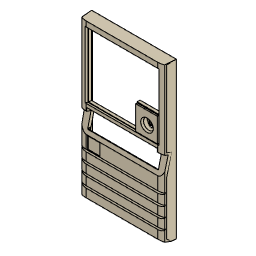
ks-330-front-1.0-dev (Autodesk Fusion 360 design; units mm, degrees)
Autodesk Fusion 360 part; units mm, degrees
sketch "Base-Front" plane through (0, 0, 0) normal (0, 1, 0) x (1, 0, 0)
  line L0 (-90, 0) -> (90, 0)
  line L1 (90, 0) -> (90, -330)
  line L2 (90, -330) -> (-90, -330)
  line L3 (-90, -330) -> (-90, 0)
  dimension "d1" = 180
  dimension "d2" = 330
  constraint horizontal L0
  constraint vertical L1
  constraint horizontal L2
  constraint vertical L3
  measures "d1" distance of L0.start L0.end
  measures "d2" distance of L0.start L2.end
extrude "Extrude1" add sketch "Base-Front" along normal blind 3.25 makes body 1
sketch "Back-OuterFrame" plane through (0, 3.25, 0) normal (0, 1, 0) x (-1, 0, 0)
  line L0 (90, 330) -> (-90, 330)
  line L1 (-90, 330) -> (-90, 0)
  line L2 (-90, 0) -> (90, 0)
  line L3 (90, 0) -> (90, 330)
  line L4 (-88, 328) -> (88, 328)
  line L5 (88, 328) -> (88, 2)
  line L6 (88, 2) -> (-88, 2)
  line L7 (-88, 2) -> (-88, 328)
  dimension "d5" = 2
  dimension "d6" = 2
  dimension "d7" = 2
  dimension "d8" = 2
  constraint horizontal L4
  constraint vertical L5
  constraint horizontal L6
  constraint vertical L7
  measures "d5" distance of L3 L5
  measures "d6" distance of L1 L7
  measures "d7" distance of L0 L4.end
  measures "d8" distance of L2 L6
sketch "Back-DriveBay" plane through (0, 3.25, 165) normal (0, 1, 0) x (-1, 0, 0)
  line L0 (-75, 153) -> (75, 153)
  line L1 (75, 153) -> (75, 14.5)
  line L2 (75, 14.5) -> (-75, 14.5)
  line L3 (-75, 14.5) -> (-75, 153)
  line L4 (-90, 165) -> (-90, -165)
  line L5 (90, -165) -> (90, 165)
  line L6 (-75, 153) -> (74.5, 153)
  line L7 (74.5, 153) -> (74.5, 109.75)
  line L8 (74.5, 109.75) -> (-75, 109.75)
  line L9 (-75, 109.75) -> (-75, 153)
  line L10 (-75, 109.75) -> (74.5, 109.75)
  line L11 (74.5, 109.75) -> (74.5, 66.5)
  line L12 (74.5, 66.5) -> (-75, 66.5)
  line L13 (-75, 66.5) -> (-75, 109.75)
  line L14 (-75, 66.5) -> (-28, 66.5)
  line L15 (-28, 66.5) -> (-28, 14.5)
  line L16 (-28, 14.5) -> (-75, 14.5)
  line L17 (-75, 14.5) -> (-75, 66.5)
  line L18 (74.5, 66.9726) -> (74.5, 40.5)
  line L19 (74.5, 40.5) -> (-28, 40.5)
  line L20 (-28, 40.5) -> (-28, 66.5)
  line L21 (-90, 165) -> (90, 165)
  dimension "d9" = 150
  dimension "d10" = 15
  dimension "d11" = 16
  dimension "d12" = 43.25
  dimension "d13" = 43.25
  dimension "d14" = 138.5
  dimension "d15" = 51.75
  dimension "d16" = 47
  dimension "d17" = 102.5
  dimension "d20" = 26
  dimension "d22" = 26
  dimension "d27" = 12
  constraint horizontal L0
  constraint vertical L1
  constraint horizontal L2
  constraint vertical L3
  constraint horizontal L6
  constraint vertical L7
  constraint horizontal L8
  constraint vertical L9
  constraint horizontal L10
  constraint vertical L11
  constraint horizontal L12
  constraint vertical L13
  constraint horizontal L14
  constraint vertical L15
  constraint horizontal L16
  constraint vertical L17
  constraint coincident L2 L15.end
  constraint vertical L18
  constraint horizontal L19
  constraint vertical L20
  measures "d9" distance of L1 L3
  measures "d10" distance of L3 L4
  measures "d12" distance of L0.start L8.end
  measures "d13" distance of L8.end L12.end
  measures "d14" distance of L2 L6
  measures "d16" distance of L15 L17
  measures "d20" distance of L14.end L19.end
  measures "d22" distance of L2 L19
  measures "d27" distance of L0 L21
sketch "Back-DriveBayFrame" plane through (0, 3.25, 165) normal (0, 1, 0) x (-1, 0, 0)
  line L0 (-79, 156) -> (79, 156)
  line L1 (79, 156) -> (79, 11.5)
  line L2 (79, 11.5) -> (-79, 11.5)
  line L3 (-79, 11.5) -> (-79, 156)
  line L4 (-75, 153) -> (74.5, 153)
  line L5 (75, 14.5) -> (-75, 14.5)
  line L6 (75, 153) -> (75, 14.5)
  line L7 (-75, 14.5) -> (-75, 153)
  line L8 (-75, 153) -> (75, 153)
  line L9 (75, 153) -> (75, 14.5)
  line L10 (75, 14.5) -> (-75, 14.5)
  line L11 (-75, 14.5) -> (-75, 153)
  line L12 (-79, 156) -> (79, 156)
  line L13 (-77, 155) -> (77, 155)
  line L14 (77, 155) -> (77, 12.5)
  line L15 (77, 12.5) -> (-30, 12.5)
  line L16 (-30, 12.5) -> (-30, 14.5)
  line L17 (-77, 155) -> (-77, 64.5)
  line L18 (-77, 64.5) -> (-75, 64.5)
  line L19 (-75, 64.5) -> (-30, 64.5)
  line L20 (-30, 64.5) -> (-30, 14.5)
  line L21 (74.5, 66.5) -> (-75, 66.5)
  line L22 (-28, 66.5) -> (-28, 14.5)
  line L23 (-75, 66.5) -> (-28, 66.5)
  line L24 (-28, 14.5) -> (75, 14.5)
  line L25 (-75, 66.5) -> (-75, 153)
  line L26 (75, 153) -> (75, 14.5)
  line L27 (-28, 66.5) -> (-28, 14.5)
  dimension "d23" = 3
  dimension "d24" = 3
  dimension "d25" = 4
  dimension "d26" = 4
  dimension "d29" = 2
  dimension "d30" = 2
  dimension "d32" = 2
  dimension "d33" = 107
  dimension "d34" = 2
  dimension "d35" = 2
  dimension "d36" = 90.5
  dimension "d39" = 2
  constraint horizontal L0
  constraint vertical L1
  constraint horizontal L2
  constraint vertical L3
  constraint horizontal L8
  constraint vertical L9
  constraint horizontal L10
  constraint vertical L11
  constraint coincident L5.start L6.end
  constraint coincident L4.start L7.end
  constraint perpendicular L3 L13
  constraint perpendicular L8 L14
  constraint perpendicular L14 L15
  constraint coincident L5 L16.end
  constraint perpendicular L5 L16
  constraint perpendicular L13 L17
  constraint coincident L7 L18.end
  constraint perpendicular L7 L18
  constraint perpendicular L11 L19
  constraint vertical L20
  constraint coincident L21.end L23.start
  constraint coincident L22.start L23.end
  constraint coincident L22.end L24.start
  constraint coincident L6.start L8.end
  measures "d23" distance of L0 L4
  measures "d24" distance of L2 L5
  measures "d25" distance of L1 L6
  measures "d26" distance of L3 L7
  measures "d29" distance of L11 L17
  measures "d30" distance of L8 L13
  measures "d32" distance of L10 L15
  measures "d33" distance of L14.end L15.end
  measures "d34" distance of L15.end L16.end
  measures "d35" distance of L6 L14
  measures "d36" distance of L13.start L17.end
  measures "d39" distance of L20 L22
sketch "Back-FrontPanel" plane through (0, 3.25, 0) normal (0, 1, 0) x (-1, 0, 0)
  line L0 (90, 330) -> (-90, 330)
  line L1 (-90, 330) -> (-90, 0)
  line L2 (-90, 0) -> (90, 0)
  line L3 (90, 0) -> (90, 330)
  line L4 (-75, 171.5) -> (75, 171.5)
  line L5 (75, 171.5) -> (75, 130.5)
  line L6 (75, 130.5) -> (-75, 130.5)
  line L7 (-75, 130.5) -> (-75, 171.5)
  circle A0 centre (74, 170.5) radius 1
  circle A1 centre (-74, 170.5) radius 1
  line L8 (75, 179.5) -> (-75, 179.5)
  dimension "d41" = 41
  dimension "d42" = 15
  dimension "d43" = 10
  dimension "d44" = 150
  dimension "d47" = 1
  dimension "d48" = 1
  dimension "d51" = 8
  constraint horizontal L4
  constraint vertical L5
  constraint horizontal L6
  constraint vertical L7
  constraint tangent L5 A0
  constraint tangent L4 A0
  constraint tangent L4 A1
  constraint tangent L7 A1
  measures "d41" distance of L4.start L6.end
  measures "d42" distance of L3 L5
  measures "d44" distance of L5 L7
  measures "d47" radius of A0
  measures "d48" radius of A1
  measures "d51" distance of L4 L8
extrude "Extrude2" add sketch "Back-DriveBayFrame" along normal blind 7 contours L4 L5 L6 L7 L8 L9 L10 L11 L13 L14 L15 L16 L17 L18 L24 L25 L26 | L5 L7 L10 L11 L19 L20 L21 L22 L23 L27 bodies 1
extrude "Extrude3" add sketch "Back-DriveBayFrame" along normal blind 2.5 bodies 1
extrude "Extrude4" cut sketch "Back-DriveBayFrame" against normal blind 3.25 contours L4 L5 L6 L7 L8 L9 L10 L11 L21 L22 L23 L24 L25 L26 L27 bodies 1
sketch "Front-DriveBayFrame" plane through (0, 0, 0) normal (0, -1, 0) x (1, 0, 0)
  line L0 (28, 231.5) -> (28, 179.5)
  line L1 (28, 179.5) -> (-75, 179.5)
  line L2 (-75, 179.5) -> (-75, 318)
  line L3 (-75, 318) -> (75, 318)
  line L4 (75, 318) -> (75, 231.5)
  line L5 (75, 231.5) -> (28, 231.5)
  line L6 (90, 330) -> (-90, 330)
  line L7 (-90, 330) -> (-90, 0)
  line L8 (-90, 0) -> (90, 0)
  line L9 (90, 0) -> (90, 330)
  line L10 (-76, 319) -> (76, 319)
  line L11 (-76, 319) -> (29, 319)
  line L12 (29, 319) -> (29, 178.5)
  line L13 (29, 178.5) -> (-76, 178.5)
  line L14 (-76, 178.5) -> (-76, 319)
  line L15 (29, 230.5) -> (76, 230.5)
  line L16 (76, 230.5) -> (76, 319)
  line L17 (76, 319) -> (29, 319)
  line L18 (76, 230.5) -> (29, 230.5)
  line L19 (29, 230.5) -> (29, 178.5)
  line L20 (29, 178.5) -> (76, 178.5)
  line L21 (76, 178.5) -> (76, 230.5)
  line L22 (75, 231.5) -> (28, 231.5)
  line L23 (28, 231.5) -> (28, 179.5)
  line L24 (75, 179.5) -> (75, 231.5)
  line L25 (75, 179.5) -> (29, 179.5312)
  dimension "d58" = 1
  dimension "d59" = 1
  dimension "d60" = 1
  dimension "d61" = 1
  dimension "d62" = 1
  dimension "d63" = 1
  constraint horizontal L10
  constraint horizontal L11
  constraint vertical L12
  constraint horizontal L13
  constraint vertical L14
  constraint horizontal L15
  constraint vertical L16
  constraint horizontal L17
  constraint horizontal L18
  constraint vertical L19
  constraint horizontal L20
  constraint vertical L21
  constraint horizontal L22
  constraint vertical L23
  constraint vertical L24
  constraint coincident L0.end L1.start
  constraint coincident L4.end L5.start
  constraint coincident L19 L25.end
  measures "d58" distance of L3 L10
  measures "d59" distance of L4 L10.end
  measures "d60" distance of L2 L10.start
  measures "d61" distance of L1 L13
  measures "d62" distance of L0 L12
  measures "d63" distance of L5 L15
extrude "Extrude5" add sketch "Back-OuterFrame" along normal blind 22.25 bodies 1
sketch "Back-OuterFrameSupport" plane through (0, 3.25, 0) normal (0, 1, 0) x (-1, 0, 0)
  line L0 (88, 2) -> (88, 328)
  line L1 (88, 328) -> (-88, 328)
  line L2 (-88, 328) -> (-88, 2)
  line L3 (-88, 2) -> (88, 2)
  line L4 (-79, 321) -> (79, 321)
  line L5 (79, 321) -> (79, 176.5)
  line L6 (79, 176.5) -> (-79, 176.5)
  line L7 (-79, 176.5) -> (-79, 321)
  line L8 (-88, 328) -> (-79, 328)
  line L9 (-79, 328) -> (-79, 2)
  line L10 (-79, 2) -> (-88, 2)
  line L11 (-88, 2) -> (-88, 328)
  line L12 (88, 328) -> (79, 328)
  line L13 (79, 328) -> (79, 2)
  line L14 (79, 2) -> (88, 2)
  line L15 (88, 2) -> (88, 328)
  dimension "d67" = 9
  dimension "d68" = 326
  dimension "d69" = 326
  dimension "d70" = 9
  constraint horizontal L8
  constraint vertical L9
  constraint horizontal L10
  constraint vertical L11
  constraint coincident L1.end L2.start
  constraint horizontal L12
  constraint vertical L13
  constraint horizontal L14
  constraint vertical L15
  constraint coincident L0.end L1.start
  measures "d67" distance of L1.end L8.end
  measures "d68" distance of L1.end L2.end
  measures "d69" distance of L0.end L0.start
  measures "d70" distance of L0.end L12.end
extrude "Extrude6" add sketch "Back-OuterFrameSupport" along normal blind 3.5 contours L0 L1 L3 L5 L12 L13 L14 L15 | L1 L2 L3 L7 L8 L9 L10 L11 bodies 1
extrude "Extrude7" cut sketch "Front-DriveBayFrame" against normal blind 4 contours L0 L1 L2 L3 L5 L10 L11 L12 L13 L14 L19 L22 L23 | L5 L12 L15 L18 L22 L24 | L3 L4 L10 L12 L15 L16 L17 L18 L24 | L12 L15 L18 L19 L20 L21 L24 L25 bodies 1
sketch "Top-RoundedFrame" plane through (0, 0, 330) normal (0, 0, 1) x (-1, 0, 0)
  line L0 (90, 0) -> (-90, 0)
  line L1 (-90, 0) -> (-90, -25.5)
  line L2 (-90, -25.5) -> (90, -25.5)
  line L3 (90, -25.5) -> (90, 0)
  line L4 (-90, 0) -> (-74, 0)
  line L5 (-74, 0) -> (-74, -4)
  line L6 (-74, -4) -> (-90, -4)
  line L7 (-90, -4) -> (-90, 0)
  line L8 (74, -25.5) -> (90, -25.5)
  line L9 (0, 0) -> (0, -25.5)
  spline S0 degree 5 poles (-90, -4) (-89.384, -3.5569) (-88.0978, -2.7325) (-86.0055, -1.6808) (-82.8833, -0.6468) (-78.3897, 0.0379) (-73.2671, 0.1203) (-67.5062, -0.3861) (-61.1528, -1.4505) (-54.2729, -3.0439) (-46.9346, -5.1472) (-40.7424, -7.2333) (-35.9338, -9.0268) (-32.6565, -10.3252) (-31, -11) knots 0 0 0 0 0 0 0.1 0.2 0.3 0.4 0.5 0.6 0.7 0.8 0.9 1 1 1 1 1 1
  line L10 (90, 0) -> (90, -25.5)
  line L11 (74, -4) -> (90, -4)
  line L12 (90, -25.5) -> (-90, -25.5)
  line L13 (74, 0) -> (74, -4)
  line L14 (-90, 0) -> (90, 0)
  spline S1 degree 5 poles (90, -4) (89.384, -3.5569) (88.0978, -2.7325) (86.0055, -1.6808) (82.8833, -0.6468) (78.3897, 0.0379) (73.2671, 0.1203) (67.5062, -0.3861) (61.1528, -1.4505) (54.2729, -3.0439) (46.9346, -5.1472) (40.7424, -7.2333) (35.9338, -9.0268) (32.6565, -10.3252) (31, -11) knots 0 0 0 0 0 0 0.1 0.2 0.3 0.4 0.5 0.6 0.7 0.8 0.9 1 1 1 1 1 1
  line L15 (-94.3724, -7.1451) -> (-85.6276, -0.8549)
  line L16 (-38.2403, -8.0503) -> (-23.7597, -13.9497)
  line L17 (94.3724, -7.1451) -> (85.6276, -0.8549)
  line L18 (38.2403, -8.0503) -> (23.7597, -13.9497)
  line L19 (90, -4) -> (90, 0)
  line L20 (90, 0) -> (74, 0)
  dimension "d75" = 16
  dimension "d76" = 4
  constraint horizontal L4
  constraint vertical L5
  constraint horizontal L6
  constraint vertical L7
  constraint coincident L0.end L1.start
  constraint horizontal L8
  constraint coincident L9.start origin
  constraint midpoint L2 L9.end
  constraint midpoint L6.end L15
  constraint midpoint S0.end L16
  constraint symmetric L0.end L9 L0.start
  constraint symmetric L1.end L9 L2.end
  constraint symmetric L2.end L9 L1.end
  constraint symmetric L4.end L9 L13.start
  constraint symmetric L5.end L9 L11.start
  constraint symmetric L6.end L9 L11.end
  constraint symmetric L0.start L9 L0.end
  constraint symmetric L9 S0.end S1.end
  constraint symmetric L9 L15.start L17.start
  constraint symmetric L9 L15.end L17.end
  constraint symmetric L9 L16.start L18.start
  constraint symmetric L9 L16.end L18.end
  measures "d75" distance of L0.end L4.end
  measures "d76" distance of L0.end L6.end
extrude "Extrude8" add sketch "Top-RoundedFrame" against normal blind 330 separate body contours L0 L3 L10 L14 S1 L19 L20 | L0 L1 L4 L7 S0 L14 makes body 2 at (-81.0778, 0.4636, 165) makes body 3 at (81.0778, 0.4636, 165)
chamfer "DriveBay-Chamfer" distance 2.5 distance2 4 2 edges at (76, 0, 248.75) (-76, 0, 248.75) measured on face at (-25.3333, 0, 59.5) measured on face at (-25.3333, 0, 59.5) on bodies 1
extrude "Extrude9" cut sketch "Back-FrontPanel" against normal blind 3.25 contours L4 L5 L6 L7 A0 A1 | A1 | A0 bodies 1
sketch "Left-FrontPanelV" plane through (-90, 0, 0) normal (-1, 0, 0) x (0, -1, 0)
  line L0 (0, 0) -> (0, 330)
  line L1 (0, 330) -> (-25.5, 330)
  line L2 (-25.5, 330) -> (-25.5, 0)
  line L3 (-25.5, 0) -> (0, 0)
  line L4 (-3.25, 171.5) -> (-3.25, 130.5)
  line L5 (-3.25, 171.5) -> (0, 171.5)
  line L6 (0, 171.5) -> (0, 130.5)
  line L7 (0, 130.5) -> (-3.25, 130.5)
  line L8 (-3.25, 130.5) -> (-3.25, 171.5)
  line L9 (0, 130.5) -> (-3.25, 130.5)
  line L10 (-3.25, 130.5) -> (-3.25, 121.5)
  line L11 (-3.25, 121.5) -> (0, 121.5)
  line L12 (0, 121.5) -> (0, 130.5)
  line L13 (-10, 164.5) -> (0, 164.5)
  line L14 (0, 164.5) -> (0, 171.5)
  line L15 (-3.25, 121.5) -> (-7, 121.5)
  line L16 (0, 164.5) -> (-9.4443, 161.5222)
  line L17 (0, 121.5) -> (-9.4443, 161.5222)
  line L18 (-7, 121.5) -> (-15.9619, 159.4779)
  line L19 (-15.9619, 159.4779) -> (-16.8231, 163.1277)
  line L20 (-16.8231, 163.1277) -> (-0.0945, 168.4022)
  line L21 (-16.8231, 163.1277) -> (-3.25, 167.4073)
  line L22 (0, 164.5) -> (0, 168.4707)
  line L23 (0, 164.5) -> (0, 168.4)
  line L24 (-0.0945, 168.4022) -> (0, 168.4)
  dimension "d85" = 3.25
  dimension "d86" = 9
  dimension "d88" = 7
  dimension "d92" = 3.75
  dimension "d93" = 10
  dimension "d94" = 3.75
  dimension "d95" = 3.75
  dimension "d96" = 17.5
  constraint parallel L0 L4
  constraint horizontal L5
  constraint vertical L6
  constraint horizontal L7
  constraint vertical L8
  constraint coincident L0 L6.end
  constraint horizontal L9
  constraint vertical L10
  constraint horizontal L11
  constraint vertical L12
  constraint horizontal L13
  constraint vertical L14
  constraint perpendicular L10 L15
  constraint parallel L17 L18
  constraint parallel L18 L19
  constraint parallel L16 L20
  constraint coincident L20 L21.end
  constraint coincident L4 L21.end
  constraint parallel L20 L21
  constraint coincident L6 L22.end
  constraint coincident L22 L23.end
  measures "d85" distance of L6.end L4.end
  measures "d86" distance of L6.end L11.end
  measures "d88" distance of L5.end L13.end
  measures "d92" distance of L10.end L15.end
  measures "d93" distance of L13.start L13.end
  measures "d94" distance of L18.end L19.end
  measures "d95" distance of L16 L20
  measures "d96" angle of L13 L16
extrude "Extrude10" cut sketch "Left-FrontPanelV" against normal blind 810 contours L0 L7 L9 L12 L17 | L0 L4 L6 L7 L8 L9 L16 L17 | L4 L8 L16 L17 bodies 1
extrude "Extrude11" add sketch "Left-FrontPanelV" against normal blind 180 contours L7 L9 L10 L11 L17 | L4 L8 L10 L15 L16 L17 L18 L19 L20 L21 | L4 L7 L8 L9 L17 | L0 L4 L6 L8 L13 L14 L20 L22 L23 L24 | L4 L8 L13 L16 bodies 1
extrude "Extrude12" cut sketch "Back-FrontPanel" along normal blind 25 contours L4 L5 L6 L7 A0 A1 bodies 1
extrude "Extrude13" cut sketch "Back-FrontPanel" against normal blind 60 contours L4 L5 L6 L7 A0 A1 bodies 1
sketch "FrontPanel-Rounded" plane through (0, -27.1588, 6.4088) normal (0, -0.973269, 0.229668) x (1, 0, 0)
  line L0 (-75, 127.4994) -> (-75, 159.3736)
  line L1 (-75, 159.3736) -> (-90, 159.3736)
  line L2 (-90, 159.3736) -> (-90, 118.2522)
  line L3 (-90, 118.2522) -> (90, 118.2522)
  line L4 (90, 118.2522) -> (90, 159.3736)
  line L5 (90, 159.3736) -> (75, 159.3736)
  line L6 (75, 159.3736) -> (75, 127.4994)
  line L7 (75, 127.4994) -> (-75, 127.4994)
  circle A0 centre (74, 128.4994) radius 1
  circle A1 centre (-74, 128.4994) radius 1
  dimension "d106" = 1
  dimension "d107" = 1
  constraint tangent L6 A0
  constraint tangent L7 A0
  constraint tangent L0 A1
  constraint tangent L7 A1
  measures "d106" radius of A0
  measures "d107" radius of A1
sketch "FrontPanel-RoundedSweep" plane through (0, 0, 130.5) normal (0, 0, 1) x (-1, 0, 0)
  line L0 (-75, -9.1238) -> (75, -9.1238)
  line L1 (75, -9.1238) -> (75, -2.1238)
  line L2 (75, -2.1238) -> (-75, -2.1238)
  line L3 (-75, -2.1238) -> (-75, -9.1238)
  line L4 (75, -2.1238) -> (75, -9.1238)
  line L5 (-75, -2.1238) -> (-75, -9.1238)
  constraint coincident L1.end L2.start
  constraint coincident L0.end L1.start
  constraint coincident L2.end L3.start
  constraint coincident L0.start L3.end
sweep "Sweep1" add profiles "FrontPanel-Rounded" path "FrontPanel-RoundedSweep" along L4 section 1 contours L0 L7 A1 bodies 1
sweep "Sweep2" add profiles "FrontPanel-Rounded" path "FrontPanel-RoundedSweep" along L5 section 1 contours L6 L7 A0 bodies 1
sketch "FrontPanel-FlattenGuides" plane through (0, -20.528, 4.8441) normal (0, 0.973269, -0.229668) x (-1, 0, 0)
  line L0 (-75, 130.107) -> (-75, 162.6308)
  line L1 (-75, 162.6308) -> (-88, 162.6308)
  line L2 (-88, 162.6308) -> (-88, 119.8599)
  line L3 (-88, 119.8599) -> (88, 119.8599)
  line L4 (88, 119.8599) -> (88, 162.6308)
  line L5 (88, 162.6308) -> (75, 162.6308)
  line L6 (75, 162.6308) -> (75, 130.107)
  arc A0 (74, 129.107) -> (75, 130.107) centre (74, 130.107) ccw
  line L7 (74, 129.107) -> (-74, 129.107)
  arc A1 (-75, 130.107) -> (-74, 129.107) centre (-74, 130.107) ccw
  line L8 (-75, 130.107) -> (-75, 119.8599)
  line L9 (-75, 119.8599) -> (75, 119.8599)
  line L10 (75, 119.8599) -> (75, 130.107)
  constraint coincident L0.start A1.start
  constraint coincident L3 L8.end
  constraint tangent A1 L8
  constraint coincident L3 L9.end
  constraint perpendicular L8 L9
  constraint coincident L6.end A0.end
  constraint tangent A0 L10
sketch "FrontPanel-Flatten" plane through (0, 0, 121.5) normal (0, 0, -1) x (1, 0, 0)
  line L0 (88, -7) -> (88, -6.75)
  line L1 (88, -6.75) -> (79, -6.75)
  line L2 (79, -6.75) -> (79, -3.25)
  line L3 (79, -3.25) -> (-79, -3.25)
  line L4 (-79, -3.25) -> (-79, -6.75)
  line L5 (-79, -6.75) -> (-88, -6.75)
  line L6 (-88, -6.75) -> (-88, -7)
  line L7 (-88, -7) -> (88, -7)
  line L8 (-74.9803, -7) -> (-74.9803, -3.25)
  line L9 (-74.9803, -7) -> (75, -7)
  line L10 (75, -3.25) -> (-74.9803, -3.25)
  line L11 (75, -10) -> (75, -7)
  line L12 (75, -3.25) -> (75, -7)
  line L13 (75, -10) -> (-75, -10)
  line L14 (-75, -10) -> (-74.9803, -7)
  constraint coincident L7 L8.start
  constraint coincident L3 L8.end
  constraint perpendicular L3 L8
  constraint coincident L7 L9.end
  constraint perpendicular L8 L9
  constraint coincident L3 L10.start
  constraint perpendicular L9 L11
  constraint perpendicular L9 L12
  constraint perpendicular L11 L13
extrude "Extrude14" cut sketch "FrontPanel-Flatten" against normal blind 10 contours L7 L9 L11 L13 L14 | L3 L7 L8 L9 L10 L12 bodies 1
sketch "VentGrid-Reinforcement" plane through (0, 3.25, 0) normal (0, 1, 0) x (-1, 0, 0)
  line L0 (79, 121.5) -> (74.9803, 121.5)
  line L1 (74.9803, 121.5) -> (74.9803, 131.2813)
  ellipse E0 centre (74, 131.4733) end of major axis (73, 131.4733) minor radius 0.9733 (74, 130.5) -> (74.9803, 131.2813) ccw
  line L2 (74, 130.5) -> (-74, 130.5)
  ellipse E1 centre (-74, 131.4733) end of major axis (-75, 131.4733) minor radius 0.9733 (-75, 131.4733) -> (-74, 130.5) ccw
  line L3 (-75, 131.4733) -> (-75, 121.5)
  line L4 (-75, 121.5) -> (-79, 121.5)
  line L5 (-79, 121.5) -> (-79, 2)
  line L6 (-79, 2) -> (79, 2)
  line L7 (79, 2) -> (79, 121.5)
  line L8 (-79, 22) -> (79, 22)
  line L9 (-90, 0) -> (90, 0)
  line L10 (-79, 27.25) -> (79, 27.25)
  line L11 (-79, 44.25) -> (79, 44.25)
  line L12 (-79, 49.5) -> (79, 49.5)
  line L13 (-79, 66.5) -> (79, 66.5)
  line L14 (79, 71.75) -> (-79, 71.75)
  line L15 (-79, 94) -> (79, 94)
  line L16 (79, 88.75) -> (-79, 88.75)
  line L17 (74, 130.5) -> (-74, 130.5)
  line L18 (-79, 24.5) -> (79, 24.5)
  line L19 (79, 46.75) -> (-79, 46.75)
  line L20 (-79, 69) -> (79, 69)
  line L21 (79, 91.25) -> (-79, 91.25)
  line L22 (-38.5, 96) -> (-35.5, 96)
  line L23 (-35.5, 96) -> (-35.5, 22)
  line L24 (-35.5, 22) -> (-38.5, 22)
  line L25 (-38.5, 22) -> (-38.5, 96)
  line L26 (-1.5, 96) -> (1.5, 96)
  line L27 (1.5, 96) -> (1.5, 22)
  line L28 (1.5, 22) -> (-1.5, 22)
  line L29 (-1.5, 22) -> (-1.5, 96)
  line L30 (35.5, 96) -> (38.5, 96)
  line L31 (38.5, 96) -> (38.5, 22)
  line L32 (38.5, 22) -> (35.5, 22)
  line L33 (35.5, 22) -> (35.5, 96)
  line L34 (-90, 330) -> (-90, 0)
  line L35 (90, 0) -> (90, 330)
  line L36 (-88, 2) -> (-88, 328)
  line L37 (88, 328) -> (88, 2)
  dimension "d122" = 22
  dimension "d123" = 5.25
  dimension "d124" = 17
  dimension "d125" = 5.25
  dimension "d126" = 17
  dimension "d127" = 5.25
  dimension "d129" = 5.25
  dimension "d130" = 17
  dimension "d131" = 21.5
  dimension "d132" = 2.75
  dimension "d133" = 2.75
  dimension "d134" = 2.75
  dimension "d135" = 2.75
  dimension "d136" = 3
  dimension "d137" = 3
  dimension "d138" = 74
  dimension "d139" = 3
  dimension "d140" = 34
  dimension "d141" = 34
  dimension "d146" = 49.5
  dimension "d147" = 49
  constraint coincident L5 L8.start
  constraint coincident L7 L8.end
  constraint perpendicular L7 L8
  constraint coincident L5 L10.start
  constraint coincident L7 L10.end
  constraint perpendicular L7 L10
  constraint coincident L5 L11.start
  constraint coincident L7 L11.end
  constraint perpendicular L7 L11
  constraint coincident L5 L12.start
  constraint coincident L7 L12.end
  constraint perpendicular L7 L12
  constraint coincident L5 L13.start
  constraint coincident L7 L13.end
  constraint perpendicular L7 L13
  constraint coincident L7 L14.start
  constraint coincident L5 L14.end
  constraint perpendicular L5 L14
  constraint coincident L5 L15.start
  constraint coincident L7 L15.end
  constraint perpendicular L7 L15
  constraint coincident L7 L16.start
  constraint coincident L5 L16.end
  constraint perpendicular L5 L16
  constraint coincident L5 L18.start
  constraint coincident L7 L18.end
  constraint perpendicular L7 L18
  constraint coincident L7 L19.start
  constraint coincident L5 L19.end
  constraint perpendicular L5 L19
  constraint coincident L5 L20.start
  constraint coincident L7 L20.end
  constraint perpendicular L7 L20
  constraint coincident L7 L21.start
  constraint coincident L5 L21.end
  constraint perpendicular L5 L21
  constraint horizontal L22
  constraint vertical L23
  constraint horizontal L24
  constraint vertical L25
  constraint coincident L8 L23.end
  constraint horizontal L26
  constraint vertical L27
  constraint horizontal L28
  constraint vertical L29
  constraint coincident L8 L27.end
  constraint horizontal L30
  constraint vertical L31
  constraint horizontal L32
  constraint vertical L33
  constraint coincident L8 L31.end
  measures "d122" distance of L8 L9
  measures "d123" distance of L8 L10
  measures "d124" distance of L10 L11
  measures "d125" distance of L11 L12
  measures "d126" distance of L12 L13
  measures "d127" distance of L13 L14
  measures "d129" distance of L15 L16
  measures "d130" distance of L14 L16
  measures "d132" distance of L15 L21
  measures "d133" distance of L14 L20
  measures "d134" distance of L12 L19
  measures "d135" distance of L10 L18
  measures "d136" distance of L22.start L22.end
  measures "d137" distance of L26.start L26.end
  measures "d138" distance of L26.start L28.end
  measures "d139" distance of L30.start L30.end
  measures "d140" distance of L23 L29
  measures "d141" distance of L27 L33
  measures "d146" distance of L25 L36
extrude "Extrude15" add sketch "VentGrid-Reinforcement" along normal blind 3.5 contours L7 L15 L21 L31 | L7 L16 L21 L31 | L15 L21 L31 L33 | L15 L30 L31 L33 | L16 L21 L31 L33 | L15 L21 L27 L33 | L7 L14 L20 L31 | L14 L16 L31 L33 | L16 L21 L27 L33 | L15 L21 L27 L29 | L15 L26 L27 L29 | L7 L13 L20 L31 | L14 L20 L31 L33 | L16 L21 L27 L29 | L15 L21 L23 L29 | L13 L20 L31 L33 | L14 L20 L27 L33 | L14 L16 L27 L29 | L16 L21 L23 L29 | L15 L21 L23 L25 | L15 L22 L23 L25 | L7 L12 L19 L31 | L12 L13 L31 L33 | L13 L20 L27 L33 | L14 L20 L27 L29 | L16 L21 L23 L25 | L5 L15 L21 L25 | L7 L11 L19 L31 | L12 L19 L31 L33 | L13 L20 L27 L29 | L14 L20 L23 L29 | L14 L16 L23 L25 | L5 L16 L21 L25 | L11 L19 L31 L33 | L12 L19 L27 L33 | L12 L13 L27 L29 | L13 L20 L23 L29 | L14 L20 L23 L25 | L7 L10 L18 L31 | L10 L11 L31 L33 | L11 L19 L27 L33 | L12 L19 L27 L29 | L13 L20 L23 L25 | L5 L14 L20 L25 | L7 L8 L18 L31 | L10 L18 L31 L33 | L11 L19 L27 L29 | L12 L19 L23 L29 | L12 L13 L23 L25 | L5 L13 L20 L25 | L8 L18 L31 L32 L33 | L10 L18 L27 L33 | L10 L11 L27 L29 | L11 L19 L23 L29 | L12 L19 L23 L25 | L8 L18 L27 L33 | L10 L18 L27 L29 | L11 L19 L23 L25 | L5 L12 L19 L25 | L8 L18 L27 L28 L29 | L10 L18 L23 L29 | L10 L11 L23 L25 | L5 L11 L19 L25 | L5 L8 L18 L25 | L8 L18 L23 L29 | L10 L18 L23 L25 | L5 L10 L18 L25 | L8 L18 L23 L24 L25 bodies 1
sketch "VentGrid-Left" plane through (-90, 0, 0) normal (-1, 0, 0) x (0, -1, 0)
  line L0 (0, 121.5) -> (-9.4443, 161.5222)
  line L1 (-9.4443, 161.5222) -> (0, 164.5)
  line L2 (0, 164.5) -> (0, 330)
  line L3 (0, 330) -> (-25.5, 330)
  line L4 (-25.5, 330) -> (-25.5, 0)
  line L5 (-25.5, 0) -> (0, 0)
  line L6 (0, 0) -> (0, 121.5)
  line L7 (0, 94) -> (-4.5, 94)
  line L8 (-4.5, 94) -> (0, 89.5)
  line L9 (0, 94) -> (0, 89.5)
  line L10 (-4.5, 71.75) -> (0, 71.75)
  line L11 (0, 71.75) -> (0, 67.25)
  line L12 (0, 67.25) -> (-4.5, 71.75)
  line L13 (0, 49.5) -> (0, 45)
  line L14 (0, 49.5) -> (-4.5, 49.5)
  line L15 (-4.5, 49.5) -> (0, 45)
  line L16 (-4.5, 27.25) -> (0, 27.25)
  line L17 (0, 27.25) -> (0, 22.75)
  line L18 (-4.5, 27.25) -> (0, 22.75)
  dimension "d153" = 4.5
  dimension "d154" = 45
  dimension "d155" = 5
  dimension "d156" = 4.5
  dimension "d158" = 45
  dimension "d159" = 4.5
  dimension "d161" = 45
  dimension "d162" = 4.5
  dimension "d164" = 45
  constraint coincident L6 L7.start
  constraint perpendicular L6 L7
  constraint coincident L6 L8.end
  constraint coincident L6 L10.end
  constraint perpendicular L6 L10
  constraint perpendicular L10 L11
  constraint coincident L6 L13.start
  constraint parallel L6 L13
  constraint perpendicular L13 L14
  constraint coincident L6 L16.end
  constraint perpendicular L6 L16
  constraint perpendicular L16 L17
  measures "d153" distance of L7.start L8.end
  measures "d154" angle of L7 L8
  measures "d156" distance of L10.end L11.end
  measures "d158" angle of L10 L12
  measures "d159" distance of L13.start L13.end
  measures "d161" angle of L14 L15
  measures "d162" distance of L16.end L17.end
  measures "d164" angle of L16 L18
extrude "Extrude17" cut sketch "VentGrid-Left" against normal blind 180 contours L6 L7 L8 L9 | L6 L10 L11 L12 | L6 L13 L14 L15 | L6 L16 L17 L18 bodies 1
extrude "Extrude16" cut sketch "VentGrid-Left" against normal blind 180 contours L6 L7 L8 L9 bodies 1
sketch "FrontPanel-Stops" plane through (0, 3.25, 0) normal (0, 1, 0) x (-1, 0, 0)
  line L0 (-79, 167.4073) -> (-75, 167.4073)
  line L1 (-75, 167.4073) -> (-75, 170.5)
  arc A0 (-74, 171.5) -> (-75, 170.5) centre (-74, 170.5) ccw
  line L2 (-74, 171.5) -> (74, 171.5)
  arc A1 (75, 170.5) -> (74, 171.5) centre (74, 170.5) ccw
  line L3 (75, 170.5) -> (75, 167.4073)
  line L4 (75, 167.4073) -> (79, 167.4073)
  line L5 (79, 167.4073) -> (79, 176.5)
  line L6 (79, 176.5) -> (-79, 176.5)
  line L7 (-79, 176.5) -> (-79, 167.4073)
  line L8 (-60, 171.5) -> (-50, 171.5)
  line L9 (-50, 171.5) -> (-50, 173.5)
  line L10 (-50, 173.5) -> (-60, 173.5)
  line L11 (-60, 173.5) -> (-60, 171.5)
  line L12 (-90, 330) -> (-90, 0)
  line L13 (35, 171.5) -> (45, 171.5)
  line L14 (45, 171.5) -> (45, 173.5)
  line L15 (45, 173.5) -> (35, 173.5)
  line L16 (35, 173.5) -> (35, 171.5)
  line L17 (90, 0) -> (90, 330)
  dimension "d169" = 10
  dimension "d170" = 2
  dimension "d171" = 40
  dimension "d172" = 10
  dimension "d173" = 2
  dimension "d174" = 55
  constraint horizontal L8
  constraint vertical L9
  constraint horizontal L10
  constraint vertical L11
  constraint coincident L2 L8.start
  constraint horizontal L13
  constraint vertical L14
  constraint horizontal L15
  constraint vertical L16
  constraint coincident L2 L13.start
  measures "d169" distance of L8.start L8.end
  measures "d170" distance of L8.start L10.end
  measures "d171" distance of L9 L12
  measures "d172" distance of L13.start L13.end
  measures "d173" distance of L13.start L15.end
  measures "d174" distance of L16 L17
extrude "Extrude18" add sketch "FrontPanel-Stops" along normal blind 5 contours L2 L8 L9 L10 L11 | L2 L13 L14 L15 L16 bodies 1
sketch "StickerHole" plane through (0, 0, 0) normal (0, -1, 0) x (1, 0, 0)
  line L0 (-90, 94) -> (90, 94)
  line L1 (90, 94) -> (90, 121.5)
  line L2 (90, 121.5) -> (-90, 121.5)
  line L3 (-90, 121.5) -> (-90, 94)
  line L4 (-73, 120.75) -> (-47, 120.75)
  line L5 (-47, 120.75) -> (-47, 94.75)
  line L6 (-47, 94.75) -> (-73, 94.75)
  line L7 (-73, 94.75) -> (-73, 120.75)
  line L8 (-75, 131.4733) -> (-75, 161.5222)
  dimension "d177" = 26
  dimension "d178" = 26
  dimension "d179" = 2
  dimension "d180" = 0.75
  dimension "d181" = 0.5
  constraint horizontal L4
  constraint vertical L5
  constraint horizontal L6
  constraint vertical L7
  measures "d177" distance of L4.start L4.end
  measures "d178" distance of L4.start L6.end
  measures "d179" distance of L7 L8
  measures "d180" distance of L2 L4
extrude "Extrude19" cut sketch "StickerHole" against normal blind 1.5 contours L4 L5 L6 L7 bodies 1
sketch "BottomAngle-Bottom" plane through (0, 0, 0) normal (0, 0, -1) x (1, 0, 0)
  line L0 (90, 0) -> (-90, 0)
  line L1 (-90, 0) -> (-90, -25.5)
  line L2 (-90, -25.5) -> (90, -25.5)
  line L3 (90, -25.5) -> (90, 0)
  line L4 (90, -25.5) -> (-90, -25.5)
  line L5 (-90, -25.5) -> (-90, -14)
  line L6 (-90, -14) -> (90, -14)
  line L7 (90, -14) -> (90, -25.5)
  dimension "d184" = 11.5
  dimension "d187" = 14
  constraint horizontal L4
  constraint vertical L5
  constraint horizontal L6
  constraint vertical L7
  constraint coincident L1 L5.end
  constraint coincident L2.end L3.start
  measures "d184" distance of L2.end L6.end
  measures "d187" distance of L0 L6
extrude "Extrude20" add sketch "BottomAngle-Bottom" against normal blind 10 contours L0 L1 L3 L6 bodies 1
chamfer "Chamfer2" distance 5 distance2 15 1 edges at (0, 0, 0) measured on face at (-30, 0, 7.5833) on bodies 1
chamfer "Chamfer3" distance 10.5 distance2 8 1 edges at (0, 14, 10) measured on face at (-26.3333, 11.5833, 10) on bodies 1
sketch "PowerButton-Front" plane through (0, 0, 0) normal (0, -1, 0) x (1, 0, 0)
  line L0 (75, 179.5) -> (75, 230.5)
  line L1 (75, 230.5) -> (29, 230.5)
  line L2 (29, 230.5) -> (29, 179.5312)
  line L3 (29, 179.5312) -> (75, 179.5)
  circle A0 centre (53, 203) radius 11.4
  dimension "d192" = 22.8
  dimension "d193" = 27.5
  dimension "d194" = 24
  dimension "d195" = 24
  measures "d192" diameter of A0
  measures "d193" distance of L1 A0.centre
  measures "d194" distance of L2 A0.centre
sketch "PowerButton-Bottom" plane through (0, 3.25, 0) normal (0, 1, 0) x (-1, 0, 0)
  line L0 (-75, 179.5) -> (-30, 179.5305)
  line L1 (-30, 179.5305) -> (-30, 229.5)
  line L2 (-30, 229.5) -> (-75, 229.5)
  line L3 (-75, 229.5) -> (-75, 179.5)
  circle A0 centre (-53, 203) radius 11.4
  circle A1 centre (-53, 203) radius 15
  dimension "d196" = 22.8
  dimension "d197" = 30
  constraint concentric A0 A1
  measures "d196" diameter of A0
  measures "d197" diameter of A1
extrude "Extrude21" add sketch "PowerButton-Bottom" along normal blind 11 contours A0 | A1 bodies 1
extrude "Extrude22" cut sketch "PowerButton-Front" against normal blind 12 contours A0 bodies 1
chamfer "Chamfer4" distance 2 distance2 4 1 edges at (42.3715, 0, 207.1224) measured on face at (52.0494, 0, 225.1227) on bodies 1
sketch "PowerButton-Holes" plane through (0, 14.25, 0) normal (0, 1, 0) x (-1, 0, 0)
  circle A0 centre (-53, 203) radius 15
  line L0 (-49.9607, 188.3111) -> (-60.6983, 215.8739)
  line L1 (-45.3017, 190.1261) -> (-56.0393, 217.6889)
  circle A1 centre (-53, 203) radius 4.25
  circle A2 centre (-53, 203) radius 6.25
  line L2 (-52.0925, 200.6705) -> (-38.3111, 206.0393)
  line L3 (-52.0925, 200.6705) -> (-65.8739, 195.3017)
  line L4 (-67.6889, 199.9607) -> (-40.1261, 210.6983)
  circle A3 centre (-53, 203) radius 7.3
  dimension "d204" = 5
  dimension "d205" = 8.5
  dimension "d206" = 2
  dimension "d207" = 2.5
  dimension "d208" = 5
  dimension "d221" = 14.6
  constraint coincident A0 L0.start
  constraint coincident A0 L1.end
  constraint coincident A0 L1.start
  constraint coincident A0 L0.end
  constraint concentric A0 A2
  constraint coincident A0 L2.end
  constraint coincident A0 L3.end
  constraint coincident A0 L4.start
  constraint coincident A0 L4.end
  constraint perpendicular L1 L4
  constraint concentric A0 A3
  measures "d204" distance of L0.start L1.start
  measures "d205" diameter of A1
  measures "d206" distance of A1 A2
  measures "d207" distance of A0.centre L2.start
  measures "d208" distance of L3 L4
  measures "d221" diameter of A3
extrude "Extrude24" cut sketch "PowerButton-Holes" against normal blind 3 contours L1 A1 L2 L4 | L1 A1 L2 | L0 L1 A1 L2 L3 | L1 A1 L4 | L0 L1 L2 L3 L4 | L0 A1 L3 | L0 L1 A1 L4 | L0 A1 L3 L4 | L0 A1 L4 bodies 1
extrude "Extrude25" add sketch "PowerButton-Holes" against normal blind 4 contours A1 A2 L2 L4 | L1 A1 A2 L2 | L0 L1 A1 A2 | L1 A1 A2 L4 | L0 A1 A2 L3 | L0 L1 A1 A2 | A1 A2 L3 L4 | L0 A1 A2 L4 bodies 1
extrude "Extrude26" cut sketch "PowerButton-Holes" against normal blind 3 contours A0 L2 L4 A3 | A0 L0 L1 A3 | A0 L0 L1 A3 | A0 L3 L4 A3 bodies 1
sketch "Top-Chamfer" plane through (0, 0, 330) normal (0, 0, 1) x (1, 0, 0)
  line L0 (-90, 0) -> (-90, 25.5)
  line L1 (-90, 25.5) -> (-87.769, 0)
  line L2 (-87.769, 0) -> (-90, 0)
  line L3 (90, 0) -> (90, 25.5)
  line L4 (90, 25.5) -> (87.769, 0)
  line L5 (87.769, 0) -> (90, 0)
  dimension "d226" = 5
  dimension "d227" = 5
  constraint vertical L0
  constraint horizontal L2
  constraint vertical L3
  constraint perpendicular L3 L5
  measures "d226" angle of L0 L1
  measures "d227" angle of L3 L4
extrude "Extrude27" add sketch "Top-Chamfer" against normal blind 330 separate body makes body 4 at (89.2563, 17, 110) makes body 5 at (-89.2563, 17, 220)
combine "Combine1" operation cut target body 1 tool bodies 4 3 2 5 keep tools result as body 6 in component "Component"
component "Component" placed x (1, 0, 0) y (0, 1, 0) z (0, 0, 1) at (0, 0, 0)
equation "d12 = ( 86.5 / 2 ) * 1 mm"
equation "d13 = ( 86.5 / 2 ) * 1 mm"
equation "d20 = ( 52 / 2 ) * 1 mm"
equation "d33 = 103 mm + 4 mm"
equation "d36 = 86.5 mm + 4 mm"
equation "d64 = 25.5 mm - 3.25 mm"
equation "d197 = 28 mm + 2 mm"
equation "d198 = 7 mm + 4 mm"
equation "d221 = ( 7.3 * 2 ) * 1 mm"
named bodies: "KS-330-Front", "Tool-Round-Front-Left", "Tool-Round-Frond-Right", "Tool-Camfer-Right", "Tool-Camfer-Left"
